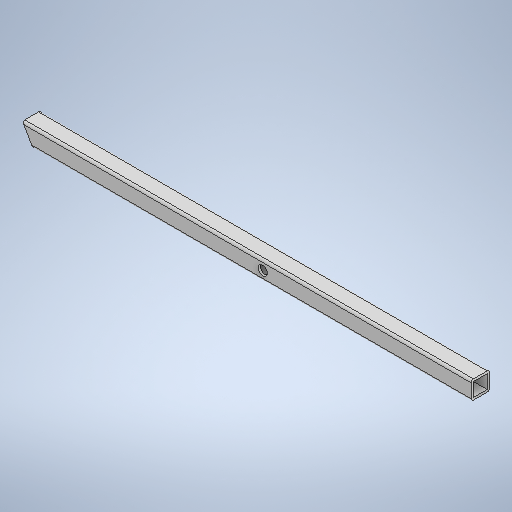
# Autodesk Inventor part: suspensionarms
Saved by Autodesk Inventor 2025.2 (Build 292293000, 293)
## iProperties
Created: 2026-03-19
Part Number: suspensionarms
Material: Generic
Document SubType Name: Modeling
Designer: hp
Density: 1 g/cm^3
Appearance: Default
Author: hp
Autodesk Inventor part; units mm, degrees
ref_plane "YZ Plane" through (0, 0, 0) normal (1, 0, 0) x (0, 1, 0)
ref_plane "XZ Plane" through (0, 0, 0) normal (0, 1, 0) x (-1, 0, 0)
ref_plane "XY Plane" through (0, 0, 0) normal (0, 0, 1) x (1, 0, 0)
sketch "Sketch1" plane through (0, 0, 0) normal (1, 0, 0) x (0, 1, 0)
  line L0 (6, 8) -> (-6, 8)
  line L1 (-8, 6) -> (-8, -6)
  line L2 (-6, -8) -> (6, -8)
  line L3 (8, -6) -> (8, 6)
  line L4 (8, 8) -> (-8, -8) construction
  line L5 (-8, 8) -> (8, -8) construction
  line L6 (6, -6) -> (-6, -6)
  line L7 (-6, -6) -> (-6, 6)
  line L8 (-6, 6) -> (6, 6)
  line L9 (6, 6) -> (6, -6)
  arc A0 (8, 6) -> (6, 8) centre (6, 6) ccw
  arc A1 (6, -8) -> (8, -6) centre (6, -6) ccw
  arc A2 (-8, -6) -> (-6, -8) centre (-6, -6) ccw
  arc A3 (-6, 8) -> (-8, 6) centre (-6, 6) ccw
  point P0 (0, 0)
  dimension "d1" = 16
  dimension "d2" = 16
  dimension "d3" = 2
  dimension "d4" = 2
  constraints: 20 end point, 8 point on circle, 8 point on line, 8 tangent, 4 centre point, 4 parallel, 3 equal radius, 2 midpoint, 2 perpendicular, 1 horizontal, 3 other
  measures "d1" distance of L5.end L4.end
  measures "d2" distance of L4.end L5.start
  measures "d3" distance between parallel lines of L2 L6
  measures "d4" radius of A0
extrude "Extrusion1" add sketch "Sketch1" along normal blind 381.62
sketch "Sketch2" plane through (0, -6, 8) normal (0, 0, 1) x (1, 0, 0)
  line L0 (0, 12) -> (0, 0) projected
  point P0 (0, 6)
  point P1 (200, 6)
  point P2 (0, 6)
  dimension "d7" = 200
  constraints: 1 midpoint
  measures "d7" distance of point (200, 6) point (0, 6)
hole "Hole1" at (200, 0, 8) direction (0, 0, -1) diameter 8 end through all
sketch "Sketch3" plane through (0, -6, 8) normal (0, 0, 1) x (1, 0, 0)
  line L0 (0, -2) -> (-9.2376, 14)
  line L1 (0, -2) -> (18.4752, -2) construction
  line L2 (-9.2376, 14) -> (0, 14)
  point P0 (0, 6)
  dimension "d15" = 120
  constraints: 6 end point, 2 horizontal, 1 equal length
  measures "d15" angle of L1 L0
ref_plane "Work Plane1" through (0, -8, 8) normal (0.8660254, 0.5, 0) x (-0.5, 0.8660254, 0)
extrude "Extrusion2" add sketch "Sketch1" against normal up to surface surface through (0, -8, 8) normal (0.8660254, 0.5, 0)
body "Solid1"
